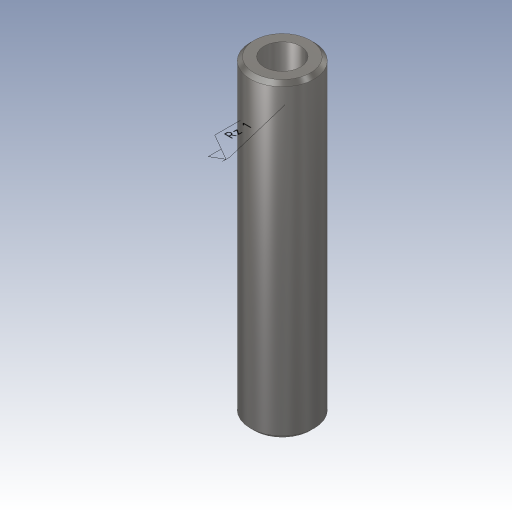
# Autodesk Inventor part: BT002_huenin20_23
Saved by Autodesk Inventor 2023.3 (Build 273359000, 359)
## iProperties
Company: HTBLA Kaindorf
RuleStatus: InUse
Created: 2023-08-12
Part Number: BT002_huenin20_23
Project: Fiberprinter-Hotend
Material: Edelstahl
Description: Heatbreak_pipe
Document SubType Name: Modeling
Designer: huenin20
Density: 8 g/cm^3
Appearance: Halbpoliert
Mass: 0.877832 g
Surface Area: 3.04017 cm^2
Volume: 0.109729 cm^3
AfterDocNew0: iProperties-Editor_aufrufen
Author: nicob
Keywords: 2023
Autodesk Inventor part; units mm, degrees
ref_plane "YZ Plane" through (0, 0, 0) normal (1, 0, 0) x (0, 1, 0)
ref_plane "XZ Plane" through (0, 0, 0) normal (0, 1, 0) x (-1, 0, 0)
ref_plane "XY Plane" through (0, 0, 0) normal (0, 0, 1) x (1, 0, 0)
sketch "Skizze3" plane through (0, 0, 0) normal (0, 0, 1) x (1, 0, 0)
  circle A0 centre (0, 0) radius 1
  circle A1 centre (0, 0) radius 1.75
  dimension "d4" = 2
  dimension "d5" = 0.75
  constraints: 2 centre point, 1 coincident
  measures "d4" diameter of A0
  measures "d5" radial gap between concentric circles of A0 A1
extrude "Extrusion3" add sketch "Skizze3" along normal blind 17
chamfer "Fase1" distance 0.2 angle 45 2 edges at (-1.75, 0, 17) (-1.75, 0, 0)
